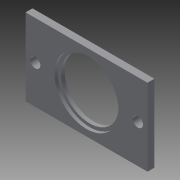
# Autodesk Inventor part: Bearing Reciver for 1-2 bearing
Saved by Autodesk Inventor 2014 SP1 (Build 180222100, 222)
## iProperties
Created: 2014-03-02
Part Number: Bearing Reciver for 1-2 bearing
Material: Generic
Document SubType Name: Modeling
Designer: Asif
Density: 1 g/cm^3
Appearance: Default
Author: Asif
Autodesk Inventor part; units mm, degrees
ref_plane "YZ Plane" through (0, 0, 0) normal (1, 0, 0) x (0, 1, 0)
ref_plane "XZ Plane" through (0, 0, 0) normal (0, 1, 0) x (-1, 0, 0)
ref_plane "XY Plane" through (0, 0, 0) normal (0, 0, 1) x (1, 0, 0)
sketch "Sketch1" plane through (0, 0, 0) normal (0, 0, 1) x (1, 0, 0)
  line L0 (0, 0) -> (60.325, 0)
  line L1 (60.325, 0) -> (60.325, 38.1)
  line L2 (60.325, 38.1) -> (0, 38.1)
  line L3 (0, 38.1) -> (0, 0)
  dimension "d0" = 60.325
  dimension "d1" = 38.1
  constraints: 8 end point, 2 parallel, 1 horizontal, 1 perpendicular
  measures "d0" distance of L0.start L0.end
  measures "d1" distance of L2.end L0.start
extrude "Extrusion1" add sketch "Sketch1" along normal blind 3.429
sketch "Sketch4" plane through (0, 0, 3.429) normal (0, 0, 1) x (1, 0, 0)
  line L0 (60.325, 38.1) -> (0, 38.1) projected
  line L1 (0, 38.1) -> (0, 0) projected
  point P0 (30.1625, 19.05)
  point P1 (30.1625, 38.1)
  point P2 (0, 19.05)
  constraints: 2 midpoint, 1 horizontal alignment, 1 vertical alignment
hole "Hole1" at (30.1625, 19.05, 3.429) direction (0, 0, -1) diameter 28.575 end through all
sketch "Sketch5" plane through (0, 0, 3.429) normal (0, 0, 1) x (1, 0, 0)
  line L0 (0, 38.1) -> (0, 0) projected
  point P0 (60.325, 0)
  point P1 (60.325, 38.1)
  point P2 (4.7752, 19.05)
  point P3 (55.5498, 19.05)
  point P4 (0, 19.05)
  point P5 (0, 19.05)
  dimension "d19" = 4.7752
  dimension "d20" = 4.7752
  dimension "d21" = 19.05
  dimension "d22" = 19.05
  constraints: 2 horizontal alignment, 2 midpoint
  measures "d19" horizontal distance of point (4.775, 19.05) L0.start
  measures "d20" horizontal distance of point (60.325, 38.1) point (55.55, 19.05)
  measures "d21" vertical distance of L0.end point (4.775, 19.05)
  measures "d22" vertical distance of point (60.325, 0) point (55.55, 19.05)
hole "Hole2" at (4.7752, 19.05, 3.429) at (55.5498, 19.05, 3.429) direction (0, 0, -1) diameter 5.1054 end through all
sketch "Sketch6" plane through (0, 0, 3.429) normal (0, 0, 1) x (1, 0, 0)
  circle A0 centre (30.1625, 19.05) radius 14.2875 projected
  circle A1 centre (30.1625, 19.05) radius 15.875
  dimension "d30" = 31.75
  constraints: 1 centre point, 1 coincident
  measures "d30" diameter of A1
extrude "Extrusion2" cut sketch "Sketch6" against normal blind 1.5875
body "Solid1"
